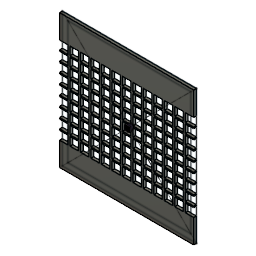
Atlas_Shelf_Master_SM001a (Autodesk Fusion 360 archive; units mm, degrees)
design "Atlas_Shelf_Master_SM001a" references "Atlas_Shelf_Corner"
part number: 2026-08-03-10-15-17-413
Autodesk Fusion 360 part; units mm, degrees
sketch "Sketch1" plane through (0, 0, 0) normal (0, 0, 1) x (1, 0, 0)
  line L0 (60.96, -60.96) -> (-60.96, -60.96)
  line L1 (-60.96, -60.96) -> (-60.96, 60.96)
  line L2 (-60.96, 60.96) -> (60.96, 60.96)
  line L3 (60.96, 60.96) -> (60.96, -60.96)
  line L4 (60.96, -60.96) -> (-60.96, 60.96) construction
  line L5 (-60.96, -60.96) -> (60.96, 60.96) construction
  line L6 (55.88, -55.88) -> (-55.88, -55.88)
  line L7 (-55.88, -55.88) -> (-55.88, 55.88)
  line L8 (-55.88, 55.88) -> (55.88, 55.88)
  line L9 (55.88, 55.88) -> (55.88, -55.88)
  line L10 (55.88, -55.88) -> (-55.88, 55.88) construction
  line L11 (-55.88, -55.88) -> (55.88, 55.88) construction
  dimension "d5" = 121.92
  dimension "d6" = 121.92
  dimension "d9" = 111.76
  dimension "d10" = 111.76
  constraint horizontal L0
  constraint perpendicular L0 L1
  constraint parallel L0 L2
  constraint parallel L1 L3
  constraint coincident L4 origin
  constraint coincident L5 origin
  constraint horizontal L6
  constraint perpendicular L6 L7
  constraint parallel L6 L8
  constraint parallel L7 L9
  constraint coincident L10 origin
  constraint coincident L11 origin
  measures "d5" distance of L1.end L2.end
  measures "d6" distance of L0.end L1.end
  measures "d9" distance of L7.end L8.end
  measures "d10" distance of L6.end L7.end
extrude "Extrude1" add sketch "Sketch1" along normal blind 2.54 contours L0 L1 L2 L3 | L6 L7 L8 L9
extrude "Extrude2" add sketch "Sketch1" along normal blind 2.54 contours L6 L7 L8 L9
sketch "Sketch2" plane through (0, 0, 2.54) normal (0, 0, 1) x (1, 0, 0)
  line L0 (3.81, 3.81) -> (-3.81, 3.81)
  line L1 (-3.81, 3.81) -> (-3.81, -3.81)
  line L2 (-3.81, -3.81) -> (3.81, -3.81)
  line L3 (3.81, -3.81) -> (3.81, 3.81)
  line L4 (3.81, 3.81) -> (-3.81, -3.81) construction
  line L5 (-3.81, 3.81) -> (3.81, -3.81) construction
  line L6 (60.96, 60.96) -> (-60.96, 60.96)
  line L7 (-60.96, 60.96) -> (-60.96, -60.96)
  line L8 (-60.96, -60.96) -> (60.96, -60.96)
  line L9 (60.96, -60.96) -> (60.96, 60.96)
  dimension "d19" = 7.62
  dimension "d20" = 7.62
  constraint horizontal L0
  constraint perpendicular L0 L1
  constraint parallel L0 L2
  constraint parallel L1 L3
  constraint coincident L4 origin
  constraint coincident L5 origin
  measures "d19" distance of L1.end L2.end
  measures "d20" distance of L0.end L1.end
extrude "Extrude3" cut sketch "Sketch2" against normal blind 7.62 contours L0 L1 L2 L3
pattern_linear "R-Pattern1" count 17 spacing 9.525 along (-1, 0, 0) both ways count 9 spacing 8.89 along (0, 1, 0) both ways of "Extrude3"
sketch "Sketch3" plane through (0, 0, 0) normal (0, 0, 1) x (1, 0, 0)
sketch "Sketch4" plane through (0, 0, 0) normal (0, 0, 1) x (1, 0, 0)
sketch "Sketch6" plane through (0, 0, 2.54) normal (0, 0, 1) x (1, 0, 0)
  line L0 (60.96, 60.96) -> (-60.96, 60.96)
  line L1 (-60.96, 31.75) -> (-60.96, 30.48)
  line L2 (-60.96, -60.96) -> (60.96, -60.96)
  line L3 (60.96, -60.96) -> (60.96, -39.37)
  line L4 (53.34, -31.75) -> (60.96, -31.75)
  line L5 (60.96, -39.37) -> (53.34, -39.37)
  line L6 (53.34, -39.37) -> (53.34, -31.75)
  line L7 (43.815, -31.75) -> (51.435, -31.75)
  line L8 (51.435, -31.75) -> (51.435, -39.37)
  line L9 (51.435, -39.37) -> (43.815, -39.37)
  line L10 (43.815, -39.37) -> (43.815, -31.75)
  line L11 (34.29, -31.75) -> (41.91, -31.75)
  line L12 (41.91, -31.75) -> (41.91, -39.37)
  line L13 (41.91, -39.37) -> (34.29, -39.37)
  line L14 (34.29, -39.37) -> (34.29, -31.75)
  line L15 (24.765, -31.75) -> (32.385, -31.75)
  line L16 (32.385, -31.75) -> (32.385, -39.37)
  line L17 (32.385, -39.37) -> (24.765, -39.37)
  line L18 (24.765, -39.37) -> (24.765, -31.75)
  line L19 (15.24, -31.75) -> (22.86, -31.75)
  line L20 (22.86, -31.75) -> (22.86, -39.37)
  line L21 (22.86, -39.37) -> (15.24, -39.37)
  line L22 (15.24, -39.37) -> (15.24, -31.75)
  line L23 (5.715, -31.75) -> (13.335, -31.75)
  line L24 (13.335, -31.75) -> (13.335, -39.37)
  line L25 (13.335, -39.37) -> (5.715, -39.37)
  line L26 (5.715, -39.37) -> (5.715, -31.75)
  line L27 (-3.81, -31.75) -> (3.81, -31.75)
  line L28 (3.81, -31.75) -> (3.81, -39.37)
  line L29 (3.81, -39.37) -> (-3.81, -39.37)
  line L30 (-3.81, -39.37) -> (-3.81, -31.75)
  line L31 (-13.335, -31.75) -> (-5.715, -31.75)
  line L32 (-5.715, -31.75) -> (-5.715, -39.37)
  line L33 (-5.715, -39.37) -> (-13.335, -39.37)
  line L34 (-13.335, -39.37) -> (-13.335, -31.75)
  line L35 (-22.86, -31.75) -> (-15.24, -31.75)
  line L36 (-15.24, -31.75) -> (-15.24, -39.37)
  line L37 (-15.24, -39.37) -> (-22.86, -39.37)
  line L38 (-22.86, -39.37) -> (-22.86, -31.75)
  line L39 (-32.385, -31.75) -> (-24.765, -31.75)
  line L40 (-24.765, -31.75) -> (-24.765, -39.37)
  line L41 (-24.765, -39.37) -> (-32.385, -39.37)
  line L42 (-32.385, -39.37) -> (-32.385, -31.75)
  line L43 (-41.91, -31.75) -> (-34.29, -31.75)
  line L44 (-34.29, -31.75) -> (-34.29, -39.37)
  line L45 (-34.29, -39.37) -> (-41.91, -39.37)
  line L46 (-41.91, -39.37) -> (-41.91, -31.75)
  line L47 (-51.435, -31.75) -> (-43.815, -31.75)
  line L48 (-43.815, -31.75) -> (-43.815, -39.37)
  line L49 (-43.815, -39.37) -> (-51.435, -39.37)
  line L50 (-51.435, -39.37) -> (-51.435, -31.75)
  line L51 (-60.96, -31.75) -> (-53.34, -31.75)
  line L52 (-53.34, -31.75) -> (-53.34, -39.37)
  line L53 (-53.34, -39.37) -> (-60.96, -39.37)
  line L54 (53.34, -22.86) -> (60.96, -22.86)
  line L55 (60.96, -30.48) -> (53.34, -30.48)
  line L56 (53.34, -30.48) -> (53.34, -22.86)
  line L57 (43.815, -22.86) -> (51.435, -22.86)
  line L58 (51.435, -22.86) -> (51.435, -30.48)
  line L59 (51.435, -30.48) -> (43.815, -30.48)
  line L60 (43.815, -30.48) -> (43.815, -22.86)
  line L61 (34.29, -22.86) -> (41.91, -22.86)
  line L62 (41.91, -22.86) -> (41.91, -30.48)
  line L63 (41.91, -30.48) -> (34.29, -30.48)
  line L64 (34.29, -30.48) -> (34.29, -22.86)
  line L65 (24.765, -22.86) -> (32.385, -22.86)
  line L66 (32.385, -22.86) -> (32.385, -30.48)
  line L67 (32.385, -30.48) -> (24.765, -30.48)
  line L68 (24.765, -30.48) -> (24.765, -22.86)
  line L69 (15.24, -22.86) -> (22.86, -22.86)
  line L70 (22.86, -22.86) -> (22.86, -30.48)
  line L71 (22.86, -30.48) -> (15.24, -30.48)
  line L72 (15.24, -30.48) -> (15.24, -22.86)
  line L73 (5.715, -22.86) -> (13.335, -22.86)
  line L74 (13.335, -22.86) -> (13.335, -30.48)
  line L75 (13.335, -30.48) -> (5.715, -30.48)
  line L76 (5.715, -30.48) -> (5.715, -22.86)
  line L77 (-3.81, -22.86) -> (3.81, -22.86)
  line L78 (3.81, -22.86) -> (3.81, -30.48)
  line L79 (3.81, -30.48) -> (-3.81, -30.48)
  line L80 (-3.81, -30.48) -> (-3.81, -22.86)
  line L81 (-13.335, -22.86) -> (-5.715, -22.86)
  line L82 (-5.715, -22.86) -> (-5.715, -30.48)
  line L83 (-5.715, -30.48) -> (-13.335, -30.48)
  line L84 (-13.335, -30.48) -> (-13.335, -22.86)
  line L85 (-22.86, -22.86) -> (-15.24, -22.86)
  line L86 (-15.24, -22.86) -> (-15.24, -30.48)
  line L87 (-15.24, -30.48) -> (-22.86, -30.48)
  line L88 (-22.86, -30.48) -> (-22.86, -22.86)
  line L89 (-32.385, -22.86) -> (-24.765, -22.86)
  line L90 (-24.765, -22.86) -> (-24.765, -30.48)
  line L91 (-24.765, -30.48) -> (-32.385, -30.48)
  line L92 (-32.385, -30.48) -> (-32.385, -22.86)
  line L93 (-41.91, -22.86) -> (-34.29, -22.86)
  line L94 (-34.29, -22.86) -> (-34.29, -30.48)
  line L95 (-34.29, -30.48) -> (-41.91, -30.48)
  line L96 (-41.91, -30.48) -> (-41.91, -22.86)
  line L97 (-51.435, -22.86) -> (-43.815, -22.86)
  line L98 (-43.815, -22.86) -> (-43.815, -30.48)
  line L99 (-43.815, -30.48) -> (-51.435, -30.48)
  line L100 (-51.435, -30.48) -> (-51.435, -22.86)
  line L101 (-60.96, -22.86) -> (-53.34, -22.86)
  line L102 (-53.34, -22.86) -> (-53.34, -30.48)
  line L103 (-53.34, -30.48) -> (-60.96, -30.48)
  line L104 (53.34, -13.97) -> (60.96, -13.97)
  line L105 (60.96, -21.59) -> (53.34, -21.59)
  line L106 (53.34, -21.59) -> (53.34, -13.97)
  line L107 (43.815, -13.97) -> (51.435, -13.97)
  line L108 (51.435, -13.97) -> (51.435, -21.59)
  line L109 (51.435, -21.59) -> (43.815, -21.59)
  line L110 (43.815, -21.59) -> (43.815, -13.97)
  line L111 (34.29, -13.97) -> (41.91, -13.97)
  line L112 (41.91, -13.97) -> (41.91, -21.59)
  line L113 (41.91, -21.59) -> (34.29, -21.59)
  line L114 (34.29, -21.59) -> (34.29, -13.97)
  line L115 (24.765, -13.97) -> (32.385, -13.97)
  line L116 (32.385, -13.97) -> (32.385, -21.59)
  line L117 (32.385, -21.59) -> (24.765, -21.59)
  line L118 (24.765, -21.59) -> (24.765, -13.97)
  line L119 (15.24, -13.97) -> (22.86, -13.97)
  line L120 (22.86, -13.97) -> (22.86, -21.59)
  line L121 (22.86, -21.59) -> (15.24, -21.59)
  line L122 (15.24, -21.59) -> (15.24, -13.97)
  line L123 (5.715, -13.97) -> (13.335, -13.97)
  line L124 (13.335, -13.97) -> (13.335, -21.59)
  line L125 (13.335, -21.59) -> (5.715, -21.59)
  line L126 (5.715, -21.59) -> (5.715, -13.97)
  line L127 (-3.81, -13.97) -> (3.81, -13.97)
  line L128 (3.81, -13.97) -> (3.81, -21.59)
  line L129 (3.81, -21.59) -> (-3.81, -21.59)
  line L130 (-3.81, -21.59) -> (-3.81, -13.97)
  line L131 (-13.335, -13.97) -> (-5.715, -13.97)
  line L132 (-5.715, -13.97) -> (-5.715, -21.59)
  line L133 (-5.715, -21.59) -> (-13.335, -21.59)
  line L134 (-13.335, -21.59) -> (-13.335, -13.97)
  line L135 (-22.86, -13.97) -> (-15.24, -13.97)
  line L136 (-15.24, -13.97) -> (-15.24, -21.59)
  line L137 (-15.24, -21.59) -> (-22.86, -21.59)
  line L138 (-22.86, -21.59) -> (-22.86, -13.97)
  line L139 (-32.385, -13.97) -> (-24.765, -13.97)
  line L140 (-24.765, -13.97) -> (-24.765, -21.59)
  line L141 (-24.765, -21.59) -> (-32.385, -21.59)
  line L142 (-32.385, -21.59) -> (-32.385, -13.97)
  line L143 (-41.91, -13.97) -> (-34.29, -13.97)
  line L144 (-34.29, -13.97) -> (-34.29, -21.59)
  line L145 (-34.29, -21.59) -> (-41.91, -21.59)
  line L146 (-41.91, -21.59) -> (-41.91, -13.97)
  line L147 (-51.435, -13.97) -> (-43.815, -13.97)
  line L148 (-43.815, -13.97) -> (-43.815, -21.59)
  line L149 (-43.815, -21.59) -> (-51.435, -21.59)
  line L150 (-51.435, -21.59) -> (-51.435, -13.97)
  line L151 (-60.96, -13.97) -> (-53.34, -13.97)
  line L152 (-53.34, -13.97) -> (-53.34, -21.59)
  line L153 (-53.34, -21.59) -> (-60.96, -21.59)
  line L154 (53.34, -5.08) -> (60.96, -5.08)
  line L155 (60.96, -12.7) -> (53.34, -12.7)
  line L156 (53.34, -12.7) -> (53.34, -5.08)
  line L157 (43.815, -5.08) -> (51.435, -5.08)
  line L158 (51.435, -5.08) -> (51.435, -12.7)
  line L159 (51.435, -12.7) -> (43.815, -12.7)
  line L160 (43.815, -12.7) -> (43.815, -5.08)
  line L161 (34.29, -5.08) -> (41.91, -5.08)
  line L162 (41.91, -5.08) -> (41.91, -12.7)
  line L163 (41.91, -12.7) -> (34.29, -12.7)
  line L164 (34.29, -12.7) -> (34.29, -5.08)
  line L165 (24.765, -5.08) -> (32.385, -5.08)
  line L166 (32.385, -5.08) -> (32.385, -12.7)
  line L167 (32.385, -12.7) -> (24.765, -12.7)
  line L168 (24.765, -12.7) -> (24.765, -5.08)
  line L169 (15.24, -5.08) -> (22.86, -5.08)
  line L170 (22.86, -5.08) -> (22.86, -12.7)
  line L171 (22.86, -12.7) -> (15.24, -12.7)
  line L172 (15.24, -12.7) -> (15.24, -5.08)
  line L173 (5.715, -5.08) -> (13.335, -5.08)
  line L174 (13.335, -5.08) -> (13.335, -12.7)
  line L175 (13.335, -12.7) -> (5.715, -12.7)
  line L176 (5.715, -12.7) -> (5.715, -5.08)
  line L177 (-3.81, -5.08) -> (3.81, -5.08)
  line L178 (3.81, -5.08) -> (3.81, -12.7)
  line L179 (3.81, -12.7) -> (-3.81, -12.7)
  line L180 (-3.81, -12.7) -> (-3.81, -5.08)
  line L181 (-13.335, -5.08) -> (-5.715, -5.08)
  line L182 (-5.715, -5.08) -> (-5.715, -12.7)
  line L183 (-5.715, -12.7) -> (-13.335, -12.7)
  line L184 (-13.335, -12.7) -> (-13.335, -5.08)
  line L185 (-22.86, -5.08) -> (-15.24, -5.08)
  line L186 (-15.24, -5.08) -> (-15.24, -12.7)
  line L187 (-15.24, -12.7) -> (-22.86, -12.7)
  line L188 (-22.86, -12.7) -> (-22.86, -5.08)
  line L189 (-32.385, -5.08) -> (-24.765, -5.08)
  line L190 (-24.765, -5.08) -> (-24.765, -12.7)
  line L191 (-24.765, -12.7) -> (-32.385, -12.7)
  line L192 (-32.385, -12.7) -> (-32.385, -5.08)
  line L193 (-41.91, -5.08) -> (-34.29, -5.08)
  line L194 (-34.29, -5.08) -> (-34.29, -12.7)
  line L195 (-34.29, -12.7) -> (-41.91, -12.7)
  line L196 (-41.91, -12.7) -> (-41.91, -5.08)
  line L197 (-51.435, -5.08) -> (-43.815, -5.08)
  line L198 (-43.815, -5.08) -> (-43.815, -12.7)
  line L199 (-43.815, -12.7) -> (-51.435, -12.7)
  line L200 (-51.435, -12.7) -> (-51.435, -5.08)
  line L201 (-60.96, -5.08) -> (-53.34, -5.08)
  line L202 (-53.34, -5.08) -> (-53.34, -12.7)
  line L203 (-53.34, -12.7) -> (-60.96, -12.7)
  line L204 (53.34, 3.81) -> (60.96, 3.81)
  line L205 (60.96, -3.81) -> (53.34, -3.81)
  line L206 (53.34, -3.81) -> (53.34, 3.81)
  line L207 (43.815, 3.81) -> (51.435, 3.81)
  line L208 (51.435, 3.81) -> (51.435, -3.81)
  line L209 (51.435, -3.81) -> (43.815, -3.81)
  line L210 (43.815, -3.81) -> (43.815, 3.81)
  line L211 (34.29, 3.81) -> (41.91, 3.81)
  line L212 (41.91, 3.81) -> (41.91, -3.81)
  line L213 (41.91, -3.81) -> (34.29, -3.81)
  line L214 (34.29, -3.81) -> (34.29, 3.81)
  line L215 (24.765, 3.81) -> (32.385, 3.81)
  line L216 (32.385, 3.81) -> (32.385, -3.81)
  line L217 (32.385, -3.81) -> (24.765, -3.81)
  line L218 (24.765, -3.81) -> (24.765, 3.81)
  line L219 (15.24, 3.81) -> (22.86, 3.81)
  line L220 (22.86, 3.81) -> (22.86, -3.81)
  line L221 (22.86, -3.81) -> (15.24, -3.81)
  line L222 (15.24, -3.81) -> (15.24, 3.81)
  line L223 (5.715, 3.81) -> (13.335, 3.81)
  line L224 (13.335, 3.81) -> (13.335, -3.81)
  line L225 (13.335, -3.81) -> (5.715, -3.81)
  line L226 (5.715, -3.81) -> (5.715, 3.81)
  line L227 (-13.335, 3.81) -> (-5.715, 3.81)
  line L228 (-5.715, 3.81) -> (-5.715, -3.81)
  line L229 (-5.715, -3.81) -> (-13.335, -3.81)
  line L230 (-13.335, -3.81) -> (-13.335, 3.81)
  line L231 (-22.86, 3.81) -> (-15.24, 3.81)
  line L232 (-15.24, 3.81) -> (-15.24, -3.81)
  line L233 (-15.24, -3.81) -> (-22.86, -3.81)
  line L234 (-22.86, -3.81) -> (-22.86, 3.81)
  line L235 (-32.385, 3.81) -> (-24.765, 3.81)
  line L236 (-24.765, 3.81) -> (-24.765, -3.81)
  line L237 (-24.765, -3.81) -> (-32.385, -3.81)
  line L238 (-32.385, -3.81) -> (-32.385, 3.81)
  line L239 (-41.91, 3.81) -> (-34.29, 3.81)
  line L240 (-34.29, 3.81) -> (-34.29, -3.81)
  line L241 (-34.29, -3.81) -> (-41.91, -3.81)
  line L242 (-41.91, -3.81) -> (-41.91, 3.81)
  line L243 (-51.435, 3.81) -> (-43.815, 3.81)
  line L244 (-43.815, 3.81) -> (-43.815, -3.81)
  line L245 (-43.815, -3.81) -> (-51.435, -3.81)
  line L246 (-51.435, -3.81) -> (-51.435, 3.81)
  line L247 (-60.96, 3.81) -> (-53.34, 3.81)
  line L248 (-53.34, 3.81) -> (-53.34, -3.81)
  line L249 (-53.34, -3.81) -> (-60.96, -3.81)
  line L250 (53.34, 12.7) -> (60.96, 12.7)
  line L251 (60.96, 5.08) -> (53.34, 5.08)
  line L252 (53.34, 5.08) -> (53.34, 12.7)
  line L253 (43.815, 12.7) -> (51.435, 12.7)
  line L254 (51.435, 12.7) -> (51.435, 5.08)
  line L255 (51.435, 5.08) -> (43.815, 5.08)
  line L256 (43.815, 5.08) -> (43.815, 12.7)
  line L257 (34.29, 12.7) -> (41.91, 12.7)
  line L258 (41.91, 12.7) -> (41.91, 5.08)
  line L259 (41.91, 5.08) -> (34.29, 5.08)
  line L260 (34.29, 5.08) -> (34.29, 12.7)
  line L261 (24.765, 12.7) -> (32.385, 12.7)
  line L262 (32.385, 12.7) -> (32.385, 5.08)
  line L263 (32.385, 5.08) -> (24.765, 5.08)
  line L264 (24.765, 5.08) -> (24.765, 12.7)
  line L265 (15.24, 12.7) -> (22.86, 12.7)
  line L266 (22.86, 12.7) -> (22.86, 5.08)
  line L267 (22.86, 5.08) -> (15.24, 5.08)
  line L268 (15.24, 5.08) -> (15.24, 12.7)
  line L269 (5.715, 12.7) -> (13.335, 12.7)
  line L270 (13.335, 12.7) -> (13.335, 5.08)
  line L271 (13.335, 5.08) -> (5.715, 5.08)
  line L272 (5.715, 5.08) -> (5.715, 12.7)
  line L273 (-3.81, 12.7) -> (3.81, 12.7)
  line L274 (3.81, 12.7) -> (3.81, 5.08)
  line L275 (3.81, 5.08) -> (-3.81, 5.08)
  line L276 (-3.81, 5.08) -> (-3.81, 12.7)
  line L277 (-13.335, 12.7) -> (-5.715, 12.7)
  line L278 (-5.715, 12.7) -> (-5.715, 5.08)
  line L279 (-5.715, 5.08) -> (-13.335, 5.08)
  line L280 (-13.335, 5.08) -> (-13.335, 12.7)
  line L281 (-22.86, 12.7) -> (-15.24, 12.7)
  line L282 (-15.24, 12.7) -> (-15.24, 5.08)
  line L283 (-15.24, 5.08) -> (-22.86, 5.08)
  line L284 (-22.86, 5.08) -> (-22.86, 12.7)
  line L285 (-32.385, 12.7) -> (-24.765, 12.7)
  line L286 (-24.765, 12.7) -> (-24.765, 5.08)
  line L287 (-24.765, 5.08) -> (-32.385, 5.08)
  line L288 (-32.385, 5.08) -> (-32.385, 12.7)
  line L289 (-41.91, 12.7) -> (-34.29, 12.7)
  line L290 (-34.29, 12.7) -> (-34.29, 5.08)
  line L291 (-34.29, 5.08) -> (-41.91, 5.08)
  line L292 (-41.91, 5.08) -> (-41.91, 12.7)
  line L293 (-51.435, 12.7) -> (-43.815, 12.7)
  line L294 (-43.815, 12.7) -> (-43.815, 5.08)
  line L295 (-43.815, 5.08) -> (-51.435, 5.08)
  line L296 (-51.435, 5.08) -> (-51.435, 12.7)
  line L297 (-60.96, 12.7) -> (-53.34, 12.7)
  line L298 (-53.34, 12.7) -> (-53.34, 5.08)
  line L299 (-53.34, 5.08) -> (-60.96, 5.08)
  line L300 (53.34, 21.59) -> (60.96, 21.59)
  line L301 (60.96, 13.97) -> (53.34, 13.97)
  line L302 (53.34, 13.97) -> (53.34, 21.59)
  line L303 (43.815, 21.59) -> (51.435, 21.59)
  line L304 (51.435, 21.59) -> (51.435, 13.97)
  line L305 (51.435, 13.97) -> (43.815, 13.97)
  line L306 (43.815, 13.97) -> (43.815, 21.59)
  line L307 (34.29, 21.59) -> (41.91, 21.59)
  line L308 (41.91, 21.59) -> (41.91, 13.97)
  line L309 (41.91, 13.97) -> (34.29, 13.97)
  line L310 (34.29, 13.97) -> (34.29, 21.59)
  line L311 (24.765, 21.59) -> (32.385, 21.59)
  line L312 (32.385, 21.59) -> (32.385, 13.97)
  line L313 (32.385, 13.97) -> (24.765, 13.97)
  line L314 (24.765, 13.97) -> (24.765, 21.59)
  line L315 (15.24, 21.59) -> (22.86, 21.59)
  line L316 (22.86, 21.59) -> (22.86, 13.97)
  line L317 (22.86, 13.97) -> (15.24, 13.97)
  line L318 (15.24, 13.97) -> (15.24, 21.59)
  line L319 (5.715, 21.59) -> (13.335, 21.59)
  line L320 (13.335, 21.59) -> (13.335, 13.97)
  line L321 (13.335, 13.97) -> (5.715, 13.97)
  line L322 (5.715, 13.97) -> (5.715, 21.59)
  line L323 (-3.81, 21.59) -> (3.81, 21.59)
  line L324 (3.81, 21.59) -> (3.81, 13.97)
  line L325 (3.81, 13.97) -> (-3.81, 13.97)
  line L326 (-3.81, 13.97) -> (-3.81, 21.59)
  line L327 (-13.335, 21.59) -> (-5.715, 21.59)
  line L328 (-5.715, 21.59) -> (-5.715, 13.97)
  line L329 (-5.715, 13.97) -> (-13.335, 13.97)
  line L330 (-13.335, 13.97) -> (-13.335, 21.59)
  line L331 (-22.86, 21.59) -> (-15.24, 21.59)
  line L332 (-15.24, 21.59) -> (-15.24, 13.97)
  line L333 (-15.24, 13.97) -> (-22.86, 13.97)
  line L334 (-22.86, 13.97) -> (-22.86, 21.59)
  line L335 (-32.385, 21.59) -> (-24.765, 21.59)
  line L336 (-24.765, 21.59) -> (-24.765, 13.97)
  line L337 (-24.765, 13.97) -> (-32.385, 13.97)
  line L338 (-32.385, 13.97) -> (-32.385, 21.59)
  line L339 (-41.91, 21.59) -> (-34.29, 21.59)
  line L340 (-34.29, 21.59) -> (-34.29, 13.97)
  line L341 (-34.29, 13.97) -> (-41.91, 13.97)
  line L342 (-41.91, 13.97) -> (-41.91, 21.59)
  line L343 (-51.435, 21.59) -> (-43.815, 21.59)
  line L344 (-43.815, 21.59) -> (-43.815, 13.97)
  line L345 (-43.815, 13.97) -> (-51.435, 13.97)
  line L346 (-51.435, 13.97) -> (-51.435, 21.59)
  line L347 (-60.96, 21.59) -> (-53.34, 21.59)
  line L348 (-53.34, 21.59) -> (-53.34, 13.97)
  line L349 (-53.34, 13.97) -> (-60.96, 13.97)
  line L350 (53.34, 30.48) -> (60.96, 30.48)
  line L351 (60.96, 22.86) -> (53.34, 22.86)
  line L352 (53.34, 22.86) -> (53.34, 30.48)
  line L353 (43.815, 30.48) -> (51.435, 30.48)
  line L354 (51.435, 30.48) -> (51.435, 22.86)
  line L355 (51.435, 22.86) -> (43.815, 22.86)
  line L356 (43.815, 22.86) -> (43.815, 30.48)
  line L357 (34.29, 30.48) -> (41.91, 30.48)
  line L358 (41.91, 30.48) -> (41.91, 22.86)
  line L359 (41.91, 22.86) -> (34.29, 22.86)
  line L360 (34.29, 22.86) -> (34.29, 30.48)
  line L361 (24.765, 30.48) -> (32.385, 30.48)
  line L362 (32.385, 30.48) -> (32.385, 22.86)
  line L363 (32.385, 22.86) -> (24.765, 22.86)
  line L364 (24.765, 22.86) -> (24.765, 30.48)
  line L365 (15.24, 30.48) -> (22.86, 30.48)
  line L366 (22.86, 30.48) -> (22.86, 22.86)
  line L367 (22.86, 22.86) -> (15.24, 22.86)
  line L368 (15.24, 22.86) -> (15.24, 30.48)
  line L369 (5.715, 30.48) -> (13.335, 30.48)
  line L370 (13.335, 30.48) -> (13.335, 22.86)
  line L371 (13.335, 22.86) -> (5.715, 22.86)
  line L372 (5.715, 22.86) -> (5.715, 30.48)
  line L373 (-3.81, 30.48) -> (3.81, 30.48)
  line L374 (3.81, 30.48) -> (3.81, 22.86)
  line L375 (3.81, 22.86) -> (-3.81, 22.86)
  line L376 (-3.81, 22.86) -> (-3.81, 30.48)
  line L377 (-13.335, 30.48) -> (-5.715, 30.48)
  line L378 (-5.715, 30.48) -> (-5.715, 22.86)
  line L379 (-5.715, 22.86) -> (-13.335, 22.86)
  line L380 (-13.335, 22.86) -> (-13.335, 30.48)
  line L381 (-22.86, 30.48) -> (-15.24, 30.48)
  line L382 (-15.24, 30.48) -> (-15.24, 22.86)
  line L383 (-15.24, 22.86) -> (-22.86, 22.86)
  line L384 (-22.86, 22.86) -> (-22.86, 30.48)
  line L385 (-32.385, 30.48) -> (-24.765, 30.48)
  line L386 (-24.765, 30.48) -> (-24.765, 22.86)
  line L387 (-24.765, 22.86) -> (-32.385, 22.86)
  line L388 (-32.385, 22.86) -> (-32.385, 30.48)
  line L389 (-41.91, 30.48) -> (-34.29, 30.48)
  line L390 (-34.29, 30.48) -> (-34.29, 22.86)
  line L391 (-34.29, 22.86) -> (-41.91, 22.86)
  line L392 (-41.91, 22.86) -> (-41.91, 30.48)
  line L393 (-51.435, 30.48) -> (-43.815, 30.48)
  line L394 (-43.815, 30.48) -> (-43.815, 22.86)
  line L395 (-43.815, 22.86) -> (-51.435, 22.86)
  line L396 (-51.435, 22.86) -> (-51.435, 30.48)
  line L397 (-60.96, 30.48) -> (-53.34, 30.48)
  line L398 (-53.34, 30.48) -> (-53.34, 22.86)
  line L399 (-53.34, 22.86) -> (-60.96, 22.86)
  line L400 (53.34, 39.37) -> (60.96, 39.37)
  line L401 (60.96, 31.75) -> (53.34, 31.75)
  line L402 (53.34, 31.75) -> (53.34, 39.37)
  line L403 (43.815, 39.37) -> (51.435, 39.37)
  line L404 (51.435, 39.37) -> (51.435, 31.75)
  line L405 (51.435, 31.75) -> (43.815, 31.75)
  line L406 (43.815, 31.75) -> (43.815, 39.37)
  line L407 (34.29, 39.37) -> (41.91, 39.37)
  line L408 (41.91, 39.37) -> (41.91, 31.75)
  line L409 (41.91, 31.75) -> (34.29, 31.75)
  line L410 (34.29, 31.75) -> (34.29, 39.37)
  line L411 (24.765, 39.37) -> (32.385, 39.37)
  line L412 (32.385, 39.37) -> (32.385, 31.75)
  line L413 (32.385, 31.75) -> (24.765, 31.75)
  line L414 (24.765, 31.75) -> (24.765, 39.37)
  line L415 (15.24, 39.37) -> (22.86, 39.37)
  line L416 (22.86, 39.37) -> (22.86, 31.75)
  line L417 (22.86, 31.75) -> (15.24, 31.75)
  line L418 (15.24, 31.75) -> (15.24, 39.37)
  line L419 (5.715, 39.37) -> (13.335, 39.37)
  line L420 (13.335, 39.37) -> (13.335, 31.75)
  line L421 (13.335, 31.75) -> (5.715, 31.75)
  line L422 (5.715, 31.75) -> (5.715, 39.37)
  line L423 (-3.81, 39.37) -> (3.81, 39.37)
  line L424 (3.81, 39.37) -> (3.81, 31.75)
  line L425 (3.81, 31.75) -> (-3.81, 31.75)
  line L426 (-3.81, 31.75) -> (-3.81, 39.37)
  line L427 (-13.335, 39.37) -> (-5.715, 39.37)
  line L428 (-5.715, 39.37) -> (-5.715, 31.75)
  line L429 (-5.715, 31.75) -> (-13.335, 31.75)
  line L430 (-13.335, 31.75) -> (-13.335, 39.37)
  line L431 (-22.86, 39.37) -> (-15.24, 39.37)
  line L432 (-15.24, 39.37) -> (-15.24, 31.75)
  line L433 (-15.24, 31.75) -> (-22.86, 31.75)
  line L434 (-22.86, 31.75) -> (-22.86, 39.37)
  line L435 (-32.385, 39.37) -> (-24.765, 39.37)
  line L436 (-24.765, 39.37) -> (-24.765, 31.75)
  line L437 (-24.765, 31.75) -> (-32.385, 31.75)
  line L438 (-32.385, 31.75) -> (-32.385, 39.37)
  line L439 (-41.91, 39.37) -> (-34.29, 39.37)
  line L440 (-34.29, 39.37) -> (-34.29, 31.75)
  line L441 (-34.29, 31.75) -> (-41.91, 31.75)
  line L442 (-41.91, 31.75) -> (-41.91, 39.37)
  line L443 (-51.435, 39.37) -> (-43.815, 39.37)
  line L444 (-43.815, 39.37) -> (-43.815, 31.75)
  line L445 (-43.815, 31.75) -> (-51.435, 31.75)
  line L446 (-51.435, 31.75) -> (-51.435, 39.37)
  line L447 (-60.96, 39.37) -> (-53.34, 39.37)
  line L448 (-53.34, 39.37) -> (-53.34, 31.75)
  line L449 (-53.34, 31.75) -> (-60.96, 31.75)
  circle A0 centre (-65.9663, 27.8788) radius 2.794
  line L450 (-60.96, 22.86) -> (-60.96, 21.59)
  line L451 (-60.96, 13.97) -> (-60.96, 12.7)
  line L452 (-60.96, 5.08) -> (-60.96, 3.81)
  line L453 (-60.96, -3.81) -> (-60.96, -5.08)
  line L454 (-60.96, -12.7) -> (-60.96, -13.97)
  line L455 (-60.96, -21.59) -> (-60.96, -22.86)
  line L456 (-60.96, -30.48) -> (-60.96, -31.75)
  line L457 (-60.96, -39.37) -> (-60.96, -60.96)
  line L458 (60.96, -31.75) -> (60.96, -30.48)
  line L459 (60.96, -22.86) -> (60.96, -21.59)
  line L460 (60.96, -13.97) -> (60.96, -12.7)
  line L461 (60.96, -5.08) -> (60.96, -3.81)
  line L462 (60.96, 3.81) -> (60.96, 5.08)
  line L463 (60.96, 12.7) -> (60.96, 13.97)
  line L464 (60.96, 21.59) -> (60.96, 22.86)
  line L465 (60.96, 30.48) -> (60.96, 31.75)
  line L466 (60.96, 39.37) -> (60.96, 60.96)
  line L467 (-60.96, 60.96) -> (-60.96, 39.37)
  line L468 (-3.81, 3.81) -> (3.81, 3.81)
  line L469 (3.81, 3.81) -> (3.81, -3.81)
  line L470 (3.81, -3.81) -> (-3.81, -3.81)
  line L471 (-3.81, -3.81) -> (-3.81, 3.81)
  point P0 (-40.64, 40.64)
  point P1 (-40.64, -40.64)
  point P2 (40.64, 40.64)
  point P3 (40.64, -40.64)
  dimension "d61" = 5.588
  measures "d61" diameter of A0
extrude "Extrude4" [rolled back] along distance -5.08 taper angle 0
extrude "Extrude5" [rolled back] along distance -5.08 taper angle 0
extrude "Extrude6" [rolled back] along distance -7.62 taper angle 0
extrude "Extrude7" [rolled back] along distance -5.08 taper angle 0
sketch "Sketch5" plane through (0, 0, 0) normal (0, 0, 1) x (1, 0, 0)
equation "shelfWidth = 4.8 in"
equation "shelfDepth = 4.8 in"
equation "shelfThickness = 0.1 in"
equation "borderWidth = 0.2 in"
equation "d5 = shelfWidth"
equation "d6 = shelfDepth"
equation "innerWidth = shelfWidth - ( 2 * borderWidth )"
equation "innerDepth = shelfDepth - ( 2 * borderWidth )"
equation "d9 = innerWidth"
equation "d10 = innerDepth"
equation "d11 = shelfThickness"
equation "d13 = shelfInnerPanelThickness"
equation "shelfInnerPanelThickness = 0.1 in"
equation "gridCutout = 0.3 in"
equation "gridWidthCount = 4 in"
equation "gridDepthCount = 3 in"
equation "d19 = gridCutout"
equation "d20 = gridCutout"
equation "pinHoldThickness = 0.03 in"
equation "pinHoleDiameter = 0.25 in - pinHoldThickness"
equation "d61 = pinHoleDiameter"

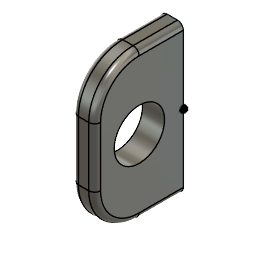
design "Atlas_ShelfTab_ST001"
part number: 2026-07-26-16-47-24-662
Autodesk Fusion 360 part; units mm, degrees
sketch "Sketch1" plane through (0, 0, 0) normal (0, 0, 1) x (1, 0, 0)
  line L0 (0.9525, 6.35) -> (-0.9525, 6.35)
  line L1 (-0.9525, 6.35) -> (-0.9525, -6.35)
  line L2 (-0.9525, -6.35) -> (0.9525, -6.35)
  line L3 (0.9525, -6.35) -> (0.9525, 6.35)
  line L4 (0.9525, 6.35) -> (-0.9525, -6.35) construction
  line L5 (-0.9525, 6.35) -> (0.9525, -6.35) construction
  dimension "d7" = 1.905
  dimension "d8" = 12.7
  constraint horizontal L0
  constraint perpendicular L0 L1
  constraint parallel L0 L2
  constraint parallel L1 L3
  constraint coincident L4 origin
  constraint coincident L5 origin
  measures "d7" distance of L1.end L2.end
  measures "d8" distance of L0.end L1.end
extrude "Extrude1" add sketch "Sketch1" along normal blind 7.62
sketch "Sketch2" plane through (0.9525, 0, 0) normal (1, 0, 0) x (0, 0, -1)
  line L0 (0, -6.35) -> (0, 6.35)
  line L1 (0, 6.35) -> (-7.62, 6.35)
  line L2 (-7.62, 6.35) -> (-7.62, -6.35)
  line L3 (-7.62, -6.35) -> (0, -6.35)
  circle A0 centre (-3.7773, 0) radius 2.159
  dimension "d11" = 4.318
  measures "d11" diameter of A0
extrude "Extrude2" cut sketch "Sketch2" against normal blind 12.7 contours A0
sketch "Sketch3" plane through (0, 0, 0) normal (0, 0, -1) x (-1, 0, 0)
  line L0 (-0.9525, 6.35) -> (-0.9525, -6.35)
  line L1 (-0.9525, -6.35) -> (0.9525, -6.35)
  line L2 (0.9525, -6.35) -> (0.9525, 6.35)
  line L3 (0.9525, 6.35) -> (-0.9525, 6.35)
  point P0 (-0.9525, 0)
  constraint midpoint L0 P0
fillet "Fillet1" radius 3.81 2 edges at (0, 6.35, 7.62) (0, -6.35, 7.62)
fillet "Fillet2" radius 0.508 10 edges at (0.9525, -6.35, 1.905) (0.9525, -5.2341, 6.5041) (0.9525, 0, 7.62) (0.9525, 5.2341, 6.5041) (0.9525, 6.35, 1.905) (-0.9525, 6.35, 1.905) (-0.9525, 5.2341, 6.5041) (-0.9525, 0, 7.62) (-0.9525, -5.2341, 6.5041) (-0.9525, -6.35, 1.905)
equation "tabHeight = 0.3 in"
equation "tabWidth = 0.5 in"
equation "tabThickness = 0.075 in"
equation "pinSize = 0.15 in"
equation "pinHoleClearance = 0.02 in"
equation "pinHoleDiameter = pinSize + pinHoleClearance"
equation "d7 = tabThickness"
equation "d8 = tabWidth"
equation "d9 = tabHeight"
equation "d11 = pinHoleDiameter"

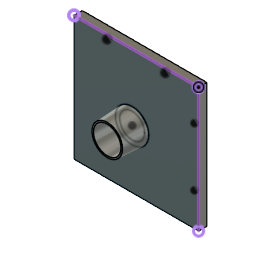
design "Atlas_Shelf_P002"
part number: 2026-07-26-17-04-48-127
Autodesk Fusion 360 part; units mm, degrees
sketch "Sketch1" plane through (0, 0, 0) normal (0, 0, 1) x (1, 0, 0)
  line L0 (19.05, -19.05) -> (-19.05, -19.05)
  line L1 (-19.05, -19.05) -> (-19.05, 19.05)
  line L2 (-19.05, 19.05) -> (19.05, 19.05)
  line L3 (19.05, 19.05) -> (19.05, -19.05)
  line L4 (19.05, -19.05) -> (-19.05, 19.05) construction
  line L5 (-19.05, -19.05) -> (19.05, 19.05) construction
  dimension "d9" = 38.1
  dimension "d10" = 38.1
  constraint horizontal L0
  constraint perpendicular L0 L1
  constraint parallel L0 L2
  constraint parallel L1 L3
  constraint coincident L4 origin
  constraint coincident L5 origin
  measures "d9" distance of L1.end L2.end
  measures "d10" distance of L0.end L1.end
extrude "Extrude1" add sketch "Sketch1" along normal blind 2.54
sketch "Sketch2" plane through (0, 0, 2.54) normal (0, 0, 1) x (1, 0, 0)
  line L0 (19.05, 19.05) -> (-19.05, 19.05)
  line L1 (-19.05, 19.05) -> (-19.05, -19.05)
  line L2 (-19.05, -19.05) -> (19.05, -19.05)
  line L3 (19.05, -19.05) -> (19.05, 19.05)
  line L4 (19.05, 19.05) -> (-19.05, 19.05)
  line L5 (19.05, -19.05) -> (19.05, 19.05)
  line L6 (-19.05, 19.05) -> (19.05, 19.05)
  line L7 (19.05, 19.05) -> (19.05, -19.05)
  circle A0 centre (-1.27, -1.27) radius 5.08
  circle A1 centre (-1.27, -1.27) radius 3.81
  point P0 (17.78, 8.89)
  point P1 (17.78, -8.89)
  dimension "d13" = 10.16
  dimension "d14" = 1.27
  dimension "d15" = 27.94
  dimension "d16" = 1.27
  dimension "d49" = 10.16
  dimension "d50" = 20.32
  dimension "d51" = 20.32
  dimension "d54" = 7.62
  constraint concentric A0 A1
  measures "d13" distance of P0 L4
  measures "d14" distance of P0 L5
  measures "d15" distance of L4 P1
  measures "d16" distance of L5 P1
  measures "d49" diameter of A0
  measures "d50" distance of L0 A0.centre
  measures "d51" distance of L5 A0.centre
  measures "d54" diameter of A1
sketch "Sketch3" plane through (0, 0, 2.54) normal (0, 0, 1) x (1, 0, 0)
  line L0 (19.05, 19.05) -> (-19.05, 19.05)
  line L1 (19.05, -19.05) -> (19.05, 19.05)
  line L2 (19.05, 19.05) -> (-19.05, 19.05)
  point P0 (8.89, 17.78)
  point P1 (-8.89, 17.78)
  dimension "d27" = 1.27
  dimension "d28" = 10.16
  dimension "d29" = 1.27
  dimension "d30" = 27.94
  measures "d27" distance of P0 L0
  measures "d28" distance of P0 L1
  measures "d29" distance of P1 L2
  measures "d30" distance of L1 P1
sketch "Sketch5" plane through (0, 0, 2.54) normal (0, 0, 1) x (1, 0, 0)
extrude "Extrude3" add sketch "Sketch2" along normal blind 7.62 draft -3 contours A0
sketch "Sketch6" plane through (0, 0, 2.54) normal (0, 0, 1) x (1, 0, 0)
  circle A0 centre (-1.27, -1.27) radius 3.1369
  point P0 (-1.27, -1.27)
  dimension "d59" = 6.2738
  constraint coincident P0 A0.centre
  measures "d59" diameter of A0
extrude "Extrude4" cut sketch "Sketch6" against normal blind 2.54
extrude "Extrude2" [suppressed]
fillet "Fillet1" [suppressed]
equation "shelfThickness = 0.1 in"
equation "shelfWidth = 1.5 in"
equation "shelfDepth = 1.5 in"
equation "trussThickness = 0.1 in"
equation "tabInset = trussThickness / 2"
equation "tabWidth = 0.5 in"
equation "tab1Offset = tabBaseOffset + tabWidth / 2"
equation "tab2Offset = tabBaseOffset + ( tabWidth / 2 ) + tabSeparation"
equation "d9 = shelfWidth"
equation "d10 = shelfDepth"
equation "d11 = shelfThickness"
equation "d13 = tab1Offset"
equation "d14 = tabInset"
equation "d15 = tab2Offset"
equation "d16 = tabInset"
equation "tabBaseOffset = 0.15 in"
equation "tabSeparation = tabWidth + 0.2 in"
equation "d27 = tabInset"
equation "d28 = tab1Offset"
equation "d29 = tabInset"
equation "d30 = tab2Offset"
equation "columnWallThickness = 0.05 in"
equation "columnClearance = 0.25 in"
equation "bossCenterOffset = 0.5 in + columnWallThickness + columnClearance"
equation "bossDiameter = 0.37 in + bossHoldThickness"
equation "bossHeight = 0.3 in"
equation "d49 = bossDiameter"
equation "d50 = bossCenterOffset"
equation "d51 = bossCenterOffset"
equation "bossWallThickness = 0.05 in"
equation "bossInnerDiameter = bossDiameter - 2 * ( bossWallThickness )"
equation "d54 = bossInnerDiameter"
equation "bossTaper = -3"
equation "d56 = bossHeight"
equation "pinHoleDiameter = 0.25 in - pinHoldThickness"
equation "d59 = pinHoleDiameter"
equation "bossHoldThickness = 0.03 in"
equation "pinHoldThickness = 0.003 in"
